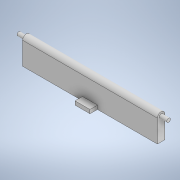
# Autodesk Inventor part: Door
Saved by Autodesk Inventor 2022 (Build 260153000, 153)
## iProperties
Created: 2021-11-11
Part Number: Door
Material: Generic
Document SubType Name: Modeling
Designer: aed0019
Density: 1 g/cm^3
Appearance: Default
Author: aed0019
Autodesk Inventor part; units mm, degrees
ref_plane "YZ Plane" through (0, 0, 0) normal (1, 0, 0) x (0, 1, 0)
ref_plane "XZ Plane" through (0, 0, 0) normal (0, 1, 0) x (-1, 0, 0)
ref_plane "XY Plane" through (0, 0, 0) normal (0, 0, 1) x (1, 0, 0)
sketch "Sketch1" plane through (0, 0, 0) normal (0, 0, 1) x (1, 0, 0)
  line L0 (-57.15, -11.1125) -> (57.15, -11.1125)
  line L1 (57.15, -11.1125) -> (57.15, 11.1125)
  line L2 (57.15, 11.1125) -> (-57.15, 11.1125)
  line L3 (-57.15, 11.1125) -> (-57.15, -11.1125)
  line L4 (-57.15, -11.1125) -> (57.15, 11.1125) construction
  line L5 (57.15, -11.1125) -> (-57.15, 11.1125) construction
  point P0 (0, 0)
  dimension "d0" = 114.3
  dimension "d14" = 22.225
  constraints: 12 end point, 2 midpoint, 2 parallel, 1 horizontal, 1 perpendicular
  measures "d0" distance of L2.end L1.end
  measures "d14" distance of L2.end L0.start
extrude "Extrusion1" add sketch "Sketch1" along normal blind 6.35
sketch "Sketch2" plane through (57.15, -11.1125, 0) normal (1, 0, 0) x (0, 0, -1)
  circle A0 centre (-3.175, 19.05) radius 1.5875
  line L0 (0, 22.225) -> (-6.35, 22.225) projected
  point P0 (0, 11.1125)
  dimension "d3" = 3.175
  dimension "d4" = 3.175
  constraints: 1 centre point
  measures "d3" diameter of A0
  measures "d4" distance from line of L0 A0.centre
extrude "Extrusion2" add sketch "Sketch2" along normal blind 6.35
sketch "Sketch3" plane through (-57.15, -11.1125, 0) normal (-1, 0, 0) x (0, 0, 1)
  circle A0 centre (3.175, 19.05) radius 1.5875 projected
  circle A1 centre (3.175, 19.05) radius 1.5875
  point P0 (0, 11.1125)
  constraints: 1 centre point, 1 coincident
extrude "Extrusion3" add sketch "Sketch3" along normal blind 6.35
sketch "Sketch4" plane through (0, 0, 6.35) normal (0, 0, 1) x (1, 0, 0)
  line L0 (-57.15, -11.1125) -> (57.15, -11.1125) projected
  line L1 (-6.35, -11.1125) -> (6.35, -11.1125)
  line L2 (6.35, -11.1125) -> (6.35, -7.9375)
  line L3 (6.35, -7.9375) -> (-6.35, -7.9375)
  line L4 (-6.35, -7.9375) -> (-6.35, -11.1125)
  line L5 (-57.15, 11.1125) -> (-57.15, -11.1125) projected
  point P0 (0, 0)
  point P1 (6.35, -11.1125)
  dimension "d9" = 12.7
  dimension "d10" = 3.175
  dimension "d11" = 50.8
  constraints: 8 end point, 2 parallel, 1 horizontal, 1 perpendicular, 1 point on line
  measures "d9" distance of L3.end L2.end
  measures "d10" distance of L2.end L1.end
  measures "d11" distance between parallel lines of L5 L4
extrude "Extrusion4" add sketch "Sketch4" along normal blind 6.35
fillet "Fillet1" radius 3.175 2 edges at (0, 11.1125, 6.35) (0, 11.1125, 0)
body "Solid1"
